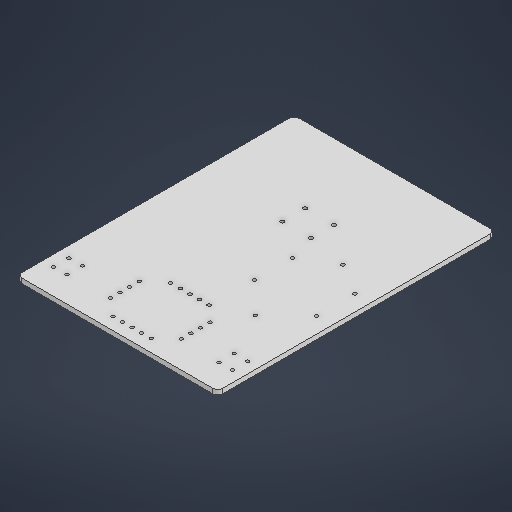
# Autodesk Inventor part: nova_base
Saved by Autodesk Inventor 2026 (Build 300175000, 175)
## iProperties
Created: 2025-03-27
Part Number: nova_base
Material: Generic
Document SubType Name: Modeling
Designer: 061210035
Density: 1 g/cm^3
Appearance: Default
Author: 061210035
Autodesk Inventor part; units mm, degrees
ref_plane "YZ Plane" through (0, 0, 0) normal (1, 0, 0) x (0, 1, 0)
ref_plane "XZ Plane" through (0, 0, 0) normal (0, 1, 0) x (-1, 0, 0)
ref_plane "XY Plane" through (0, 0, 0) normal (0, 0, 1) x (1, 0, 0)
sketch "Sketch1" plane through (0, 0, 0) normal (0, 1, 0) x (-1, 0, 0)
  line L0 (0, 0) -> (210, 0)
  line L1 (210, 0) -> (210, -290)
  line L2 (210, -290) -> (0, -290)
  line L3 (0, -290) -> (0, 0)
  dimension "d0" = 210
  dimension "d1" = 290
  constraints: 8 end point, 2 parallel, 1 horizontal, 1 perpendicular
  measures "d0" distance of L1.end L2.end
  measures "d1" distance of L0.end L1.end
extrude "Extrusion1" add sketch "Sketch1" along normal mid plane 5
fillet "Fillet1" radius 5 4 edges at (-210, 0, 0) (0, 0, 0) (0, 0, -290) (-210, 0, -290)
sketch "Sketch3" plane through (0, 2.5, 0) normal (0, 1, 0) x (1, 0, 0)
  line L0 (-105, 318.2465) -> (-105, -30.4668)
  line L1 (0, 5) -> (0, 285) projected
  line L2 (-241.3293, 200) -> (141.5713, 200)
  line L3 (-205, 0) -> (-5, 0) projected
  line L4 (-124, 216) -> (-86, 216)
  line L5 (-86, 216) -> (-86, 184)
  line L6 (-86, 184) -> (-124, 184)
  line L7 (-124, 184) -> (-124, 216)
  circle A0 centre (-90, 187.5) radius 2
  circle A1 centre (-120, 187.5) radius 2
  circle A2 centre (-90, 211.5) radius 2
  circle A3 centre (-120, 211.5) radius 2
  point P0 (0, 0)
  dimension "d20" = 105
  dimension "d21" = 200
  dimension "d22" = 38
  dimension "d23" = 32
  dimension "d24" = 19
  dimension "d25" = 16
  dimension "d26" = 4
  dimension "d27" = 1.5
  dimension "d28" = 2
  dimension "d31" = 30
  dimension "d34" = 24
  constraints: 12 end point, 4 centre point, 3 horizontal, 2 parallel, 2 vertical, 1 perpendicular, 6 other
  measures "d20" distance between parallel lines of L1 L0
  measures "d21" distance between parallel lines of L3 L2
  measures "d22" distance of L4.start L4.end
  measures "d23" distance of L4.end L5.end
  measures "d24" distance between parallel lines of L0 L7
  measures "d25" distance between parallel lines of L2 L4
  measures "d26" diameter of A0
  measures "d27" distance edge to line of A0 L6
  measures "d28" distance edge to line of A0 L5
  measures "d31" distance of A0.centre A1.centre
  measures "d34" distance of A0.centre A2.centre
extrude "Extrusion3" cut sketch "Sketch3" against normal blind 11 contours A0 | A1 | A2 | A3
sketch "Sketch7" plane through (0, 2.5, 0) normal (0, 1, 0) x (1, 0, 0)
  line L0 (-218.7677, 26.75) -> (12.5844, 26.75)
  line L1 (-205, 0) -> (-5, 0) projected
  line L2 (-11.5, -8.2138) -> (-11.5, 118.2884)
  line L3 (0, 5) -> (0, 285) projected
  circle A0 centre (-11.5, 26.75) radius 1.75
  circle A1 centre (-11.5, 42.75) radius 1.75
  circle A2 centre (-25.5, 26.75) radius 1.75
  circle A3 centre (-25.5, 42.75) radius 1.75
  line L4 (-105, -15.1628) -> (-105, 162.668)
  circle A4 centre (-198.5, 26.75) radius 1.75
  circle A5 centre (-198.5, 42.75) radius 1.75
  circle A6 centre (-184.5, 26.75) radius 1.75
  circle A7 centre (-184.5, 42.75) radius 1.75
  point P0 (0, 0)
  dimension "d45" = 26.75
  dimension "d46" = 11.5
  dimension "d47" = 3.5
  dimension "d50" = 16
  dimension "d53" = 14
  dimension "d56" = 105
  constraints: 8 centre point, 6 end point, 4 symmetric about line, 3 vertical, 2 horizontal, 2 point on line, 10 other
  measures "d45" distance between parallel lines of L1 L0
  measures "d46" distance between parallel lines of L3 L2
  measures "d47" diameter of A0
  measures "d50" distance of A0.centre A1.centre
  measures "d53" distance of A0.centre A2.centre
  measures "d56" distance between parallel lines of L3 L4
extrude "Extrusion6" cut sketch "Sketch7" against normal through all contours A4 L0 | A1 L2 | L2 A1 | A6 L0 | L0 A6 | L0 A4 | A2 L0 | L0 A2 | A0 L2 L0 | L0 L2 A0 | L2 L0 A0 | L2 A0 L0 | A3 | A5 | A7
sketch "Sketch8" plane through (0, 2.5, 0) normal (0, 1, 0) x (1, 0, 0)
  circle A0 centre (-66.5, 58.387) radius 1.75
  line L0 (0, 5) -> (0, 285) projected
  circle A1 centre (-140.5, 58.387) radius 1.75
  circle A2 centre (-66.5, 48.387) radius 1.75
  circle A3 centre (-66.5, 38.387) radius 1.75
  circle A4 centre (-66.5, 28.387) radius 1.75
  circle A5 centre (-140.5, 48.387) radius 1.75
  circle A6 centre (-140.5, 38.387) radius 1.75
  circle A7 centre (-140.5, 28.387) radius 1.75
  circle A8 centre (-122.569, 73.5) radius 1.75
  line L1 (-205, 0) -> (-5, 0) projected
  circle A9 centre (-112.569, 73.5) radius 1.75
  circle A10 centre (-102.569, 73.5) radius 1.75
  circle A11 centre (-92.569, 73.5) radius 1.75
  circle A12 centre (-82.569, 73.5) radius 1.75
  circle A13 centre (-122.569, 13) radius 1.75
  circle A14 centre (-112.569, 13) radius 1.75
  circle A15 centre (-102.569, 13) radius 1.75
  circle A16 centre (-92.569, 13) radius 1.75
  circle A17 centre (-82.569, 13) radius 1.75
  point P0 (0, 0)
  dimension "d59" = 3.5
  dimension "d60" = 66.5
  dimension "d61" = 3.5
  dimension "d62" = 74
  dimension "d70" = 10
  dimension "d74" = 10
  dimension "d79" = 3.5
  dimension "d80" = 73.5
  dimension "d83" = 10
  dimension "d88" = 3.5
  dimension "d89" = 13
  dimension "d92" = 10
  constraints: 18 centre point, 2 horizontal, 2 vertical, 1 horizontal alignment, 28 other
  measures "d59" diameter of A0
  measures "d60" distance from line of L0 A0.centre
  measures "d61" diameter of A1
  measures "d62" distance of A1.centre A0.centre
  measures "d70" distance of A0.centre A2.centre
  measures "d74" distance of A1.centre A5.centre
  measures "d79" diameter of A8
  measures "d80" distance from line of L1 A8.centre
  measures "d83" distance of A8.centre A9.centre
  measures "d88" diameter of A13
  measures "d89" distance from line of L1 A13.centre
  measures "d92" distance of A13.centre A14.centre
extrude "Extrusion7" cut sketch "Sketch8" against normal through all
sketch "Sketch9" plane through (0, 2.5, 0) normal (0, 1, 0) x (1, 0, 0)
  circle A0 centre (-16.5, 160) radius 1.75
  line L0 (0, 5) -> (0, 285) projected
  line L1 (-205, 0) -> (-5, 0) projected
  circle A1 centre (-81.5, 160) radius 1.75
  circle A2 centre (-16.5, 120) radius 1.75
  circle A3 centre (-81.5, 120) radius 1.75
  circle A4 centre (-49, 180) radius 1.75
  circle A5 centre (-49, 88.25) radius 1.75
  point P0 (0, 0)
  dimension "d97" = 3.5
  dimension "d98" = 16.5
  dimension "d101" = 160
  dimension "d104" = 65
  dimension "d107" = 40
  dimension "d110" = 3.5
  dimension "d112" = 32.5
  dimension "d113" = 180
  dimension "d114" = 3.5
  dimension "d115" = 88.25
  constraints: 6 centre point, 1 horizontal, 1 vertical, 6 other
  measures "d97" diameter of A0
  measures "d98" distance from line of L0 A0.centre
  measures "d101" distance from line of L1 A0.centre
  measures "d104" distance of A0.centre A1.centre
  measures "d107" distance of A0.centre A2.centre
  measures "d110" diameter of A4
  measures "d112" horizontal distance of A4.centre A0.centre
  measures "d113" distance from line of L1 A4.centre
  measures "d114" diameter of A5
  measures "d115" distance from line of L1 A5.centre
extrude "Extrusion8" cut sketch "Sketch9" against normal through all
equation "\"d24\" = 0.5 * d22"
equation "\"d25\" = 0.5 * d23"
equation "\"d112\" = 0.5 * d104"
body "Solid1"
